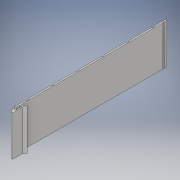
# Autodesk Inventor part: sideFold
Saved by Autodesk Inventor 2019 (Build 230136000, 136)
## iProperties
Created: 2018-07-17
Part Number: sideFold
Material: Generic
Document SubType Name: Modeling
Designer: Ge Shi
Density: 1 g/cm^3
Appearance: Default
width: 25.000 mm
length: 40.000 mm
thickness: 1.500 mm
tolerance: 0.100 mm
Author: Ge Shi
Autodesk Inventor part; units mm, degrees
ref_plane "YZ Plane" through (0, 0, 0) normal (1, 0, 0) x (0, 1, 0)
ref_plane "XZ Plane" through (0, 0, 0) normal (0, 1, 0) x (-1, 0, 0)
ref_plane "XY Plane" through (0, 0, 0) normal (0, 0, 1) x (1, 0, 0)
sketch "Sketch3" plane through (0, 0, 0) normal (0, 1, 0) x (-1, 0, 0)
  line L0 (0, 0) -> (1.5, 0)
  line L1 (1.5, 0) -> (1.5, -9.5453)
  arc A0 (0.9057, -11.4965) -> (1.5, -9.5453) centre (-2, -9.5453) ccw
  arc A1 (0.9057, -11.4965) -> (0.9057, -13.5035) centre (2.4, -12.5) ccw
  arc A2 (1.5, -15.4547) -> (0.9057, -13.5035) centre (-2, -15.4547) ccw
  line L2 (1.5, -15.4547) -> (1.5, -25)
  line L3 (1.5, -25) -> (0, -25)
  line L4 (0, -25) -> (0, 0)
  line L5 (0.6, -20.649) -> (0.6, -13.905) construction
  line L6 (0, -50) -> (1.5, -50)
  line L7 (1.5, -50) -> (1.5, -40.4547)
  arc A3 (1.5, -40.4547) -> (0.9057, -38.5035) centre (-2, -40.4547) ccw
  arc A4 (0.9057, -36.4965) -> (0.9057, -38.5035) centre (2.4, -37.5) ccw
  arc A5 (0.9057, -36.4965) -> (1.5, -34.5453) centre (-2, -34.5453) ccw
  line L8 (1.5, -34.5453) -> (1.5, -25)
  line L9 (0, -25) -> (0, -50)
  line L10 (0, -100) -> (1.5, -100)
  line L11 (1.5, -100) -> (1.5, -90.4547)
  arc A6 (1.5, -90.4547) -> (0.9057, -88.5035) centre (-2, -90.4547) ccw
  arc A7 (0.9057, -86.4965) -> (0.9057, -88.5035) centre (2.4, -87.5) ccw
  arc A8 (0.9057, -86.4965) -> (1.5, -84.5453) centre (-2, -84.5453) ccw
  line L12 (1.5, -84.5453) -> (1.5, -75)
  line L13 (1.5, -75) -> (0, -75)
  line L14 (1.5, -65.4547) -> (1.5, -75)
  line L15 (0, -75) -> (0, -50)
  arc A9 (1.5, -65.4547) -> (0.9057, -63.5035) centre (-2, -65.4547) ccw
  arc A10 (0.9057, -61.4965) -> (0.9057, -63.5035) centre (2.4, -62.5) ccw
  arc A11 (0.9057, -61.4965) -> (1.5, -59.5453) centre (-2, -59.5453) ccw
  line L16 (1.5, -50) -> (1.5, -59.5453)
  line L17 (1.5, 0) -> (1.5, 9.5453)
  arc A12 (1.5, 9.5453) -> (0.9057, 11.4965) centre (-2, 9.5453) ccw
  arc A13 (0.9057, 13.5035) -> (0.9057, 11.4965) centre (2.4, 12.5) ccw
  arc A14 (0.9057, 13.5035) -> (1.5, 15.4547) centre (-2, 15.4547) ccw
  line L18 (1.5, 15.4547) -> (1.5, 25)
  line L19 (1.5, 25) -> (0, 25)
  line L20 (0, 25) -> (0, 0)
  line L21 (1.5, 34.5453) -> (1.5, 25)
  line L22 (0, 25) -> (0, 50)
  arc A15 (1.5, 34.5453) -> (0.9057, 36.4965) centre (-2, 34.5453) ccw
  arc A16 (0.9057, 38.5035) -> (0.9057, 36.4965) centre (2.4, 37.5) ccw
  arc A17 (0.9057, 38.5035) -> (1.5, 40.4547) centre (-2, 40.4547) ccw
  line L23 (1.5, 50) -> (1.5, 40.4547)
  line L24 (0, 50) -> (1.5, 50)
  line L25 (-2.0044, 45) -> (-3.9497, 43.0546)
  line L26 (-3.9497, 43.0546) -> (-5.1305, 44.2354)
  line L27 (-5.1305, 44.2354) -> (-3.0594, 46.3065)
  line L28 (-3.0594, 46.3065) -> (-3.0594, 56.5)
  line L29 (-3.0594, 56.5) -> (-1.5594, 56.5)
  line L30 (-1.5594, 56.5) -> (0.75, 52.5)
  line L31 (0.75, 52.5) -> (-2.0594, 52.5)
  line L32 (-2.0594, 52.5) -> (-2.0594, 46.7978)
  line L33 (-2.0044, 45) -> (-0.7683, 45)
  arc A18 (0, 44.4228) -> (-0.7683, 45) centre (-0.7683, 44.2) ccw
  line L34 (-1.2, 46) -> (-0.7656, 46)
  arc A19 (-0.7656, 46) -> (0, 47.0321) centre (-0.7656, 46.8) ccw
  arc A20 (-2.0594, 46.7978) -> (-1.2, 46) centre (-1.2594, 46.7978) ccw
  line L35 (0.75, -97.4) -> (0, -96.101)
  line L36 (0, -97.4) -> (0.75, -97.4)
  line L37 (0, -75) -> (0, -96.101)
  line L38 (0, -97.4) -> (0, -100)
  point P0 (0.6, -12.5)
  dimension "d0" = 1.8
  dimension "d1" = 3.5
  dimension "d2" = 3.5
  dimension "d3" = 0.6
  dimension "d6" = 12.5
  dimension "d7" = 12.5
  dimension "d8" = 1.5
  dimension "d12" = 1
  dimension "d13" = 1
  dimension "d14" = 0.8
  dimension "d15" = 0.8
  dimension "d16" = 0.8
  dimension "d17" = 135
  dimension "d18" = 135
  dimension "d20" = 1.5
  dimension "d21" = 2.5
  dimension "d22" = 60
  dimension "d23" = 4
  dimension "d24" = 4
  dimension "d28" = 0.75
  dimension "d29" = 0.75
  dimension "d30" = 60
  dimension "d31" = 2.6
  constraints: 78 end point, 45 symmetric about line, 41 point on circle, 20 centre point, 15 point on line, 6 perpendicular, 5 tangent, 4 horizontal, 2 vertical, 1 parallel, 22 other
  measures "d1" radius of A2
  measures "d2" radius of A0
  measures "d3" distance between parallel lines of L4 L5
  measures "d6" distance from line of L0 point (0.6, -12.5)
  measures "d7" distance from line of L3 point (0.6, -12.5)
  measures "d8" distance between parallel lines of L4 L2
  measures "d12" distance between parallel lines of L34 L33
  measures "d13" distance between parallel lines of L28 L32
  measures "d14" radius of A19
  measures "d15" radius of A18
  measures "d16" radius of A20
  measures "d17" angle of L28 L27
  measures "d18" angle of L33 L25
  measures "d20" distance of L28.end L29.end
  measures "d21" distance between parallel lines of L31 L24
  measures "d22" angle of L30 L31
  measures "d23" distance between parallel lines of L31 L29
  measures "d24" distance between parallel lines of L24 L34
  measures "d28" distance from line of L23 L30.end
  measures "d29" distance from line of L11 L35.start
  measures "d30" angle of L36 L35
  measures "d31" distance between parallel lines of L10 L36
extrude "Extrusion1" add sketch "Sketch3" along normal blind 40
equation "\"d6\" = 0.5 * width"
equation "\"d7\" = 0.5 * width"
equation "\"d8\" = thickness"
equation "\"d28\" = 0.5 * thickness"
equation "\"d29\" = 0.5 * thickness"
equation "\"d31\" = d21 + tolerance"
equation "\"d9\" = length"
equation "\"width\" = 25"
equation "\"length\" = 40"
equation "\"thickness\" = 1.5"
equation "\"tolerance\" = 0.1"
body "Solid1"
